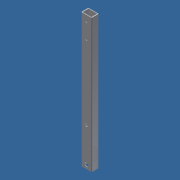
# Autodesk Inventor part: Ramie
Saved by Autodesk Inventor 2014 SP1 (Build 180222100, 222)
## iProperties
Created: 2014-09-01
Part Number: Ramie
Material: Aluminium 6061
Document SubType Name: Modeling
Designer: Marcin
Density: 2.71 g/cm^3
Appearance: Aluminium - płaski
Author: Marcin
Autodesk Inventor part; units mm, degrees
ref_plane "YZ Plane" through (0, 0, 0) normal (1, 0, 0) x (0, 1, 0)
ref_plane "XZ Plane" through (0, 0, 0) normal (0, 1, 0) x (-1, 0, 0)
ref_plane "XY Plane" through (0, 0, 0) normal (0, 0, 1) x (1, 0, 0)
sketch "Szkic1" plane through (0, 0, 0) normal (0, 0, 1) x (1, 0, 0)
  line L0 (-6.85, 5.35) -> (6.85, 5.35)
  line L1 (7.85, 4.35) -> (7.85, -4.35)
  line L2 (6.85, -5.35) -> (-6.85, -5.35)
  line L3 (-7.85, -4.35) -> (-7.85, 4.35)
  line L4 (-7.85, 5.35) -> (7.85, -5.35) construction
  line L5 (7.85, 5.35) -> (-7.85, -5.35) construction
  line L6 (-6.45, 4.3959) -> (6.45, 4.3959)
  line L7 (6.45, 4.3959) -> (6.45, -4.3959)
  line L8 (6.45, -4.3959) -> (-6.45, -4.3959)
  line L9 (-6.45, -4.3959) -> (-6.45, 4.3959)
  line L10 (-6.45, 4.3959) -> (6.45, -4.3959) construction
  line L11 (6.45, 4.3959) -> (-6.45, -4.3959) construction
  arc A0 (-6.85, 5.35) -> (-7.85, 4.35) centre (-6.85, 4.35) ccw
  arc A1 (-7.85, -4.35) -> (-6.85, -5.35) centre (-6.85, -4.35) ccw
  arc A2 (6.85, -5.35) -> (7.85, -4.35) centre (6.85, -4.35) ccw
  arc A3 (7.85, 4.35) -> (6.85, 5.35) centre (6.85, 4.35) ccw
  point P0 (0, 0)
  dimension "d0" = 10.7
  dimension "d1" = 15.7
  dimension "d2" = 1.4
  dimension "d3" = 1
  constraints: 24 end point, 9 point on line, 8 point on circle, 8 tangent, 4 centre point, 4 midpoint, 4 parallel, 3 equal radius, 2 horizontal, 2 perpendicular
  measures "d0" distance between parallel lines of L2 L0
  measures "d1" distance between parallel lines of L1 L3
  measures "d2" distance between parallel lines of L1 L7
  measures "d3" radius of A0
extrude "Wyciągnięcie proste1" add sketch "Szkic1" along normal blind 200
sketch "Szkic2" plane through (-6.85, 5.35, 0) normal (0, 1, 0) x (1, 0, 0)
  point P0 (6.882, -6)
hole "Otwór1" at (0.032, 5.35, 6) direction (0, -1, 0) diameter 6 depth 0.9541
sketch "Szkic3" plane through (-6.45, -4.3959, 0) normal (0, 1, 0) x (1, 0, 0)
  point P0 (6.482, -6)
hole "Otwór2" at (0.032, -4.3959, 6) direction (0, -1, 0) diameter 6 depth 0.9541
sketch "Szkic4" plane through (-6.85, 5.35, 0) normal (0, 1, 0) x (1, 0, 0)
  point P0 (6.882, -57)
hole "Otwór3" at (0.032, 5.35, 57) direction (0, -1, 0) diameter 4.5 depth 0.9541
sketch "Szkic5" plane through (-6.45, -4.3959, 0) normal (0, 1, 0) x (1, 0, 0)
  point P0 (6.482, -57)
hole "Otwór4" at (0.032, -4.3959, 57) direction (0, -1, 0) diameter 4.5 depth 0.9541
sketch "Szkic6" plane through (-6.85, 5.35, 0) normal (0, 1, 0) x (1, 0, 0)
  point P0 (6.85, -191.6)
hole "Otwór5" at (0, 5.35, 191.6) direction (0, -1, 0) diameter 3.5 depth 0.9541
sketch "Szkic7" plane through (-6.85, -5.35, 0) normal (0, -1, 0) x (1, 0, 0)
  point P0 (6.85, 191.6)
hole "Otwór6" at (0, -5.35, 191.6) direction (0, 1, 0) diameter 3.5 depth 0.9541
sketch "Szkic8" plane through (-6.85, 5.35, 0) normal (0, 1, 0) x (1, 0, 0)
  point P0 (6.85, -168.4)
hole "Otwór7" at (0, 5.35, 168.4) direction (0, -1, 0) diameter 3.5 depth 0.9541
sketch "Szkic9" plane through (-6.85, -5.35, 0) normal (0, -1, 0) x (1, 0, 0)
  point P0 (6.85, 168.4)
hole "Otwór8" at (0, -5.35, 168.4) direction (0, 1, 0) diameter 3.5 depth 0.9541
